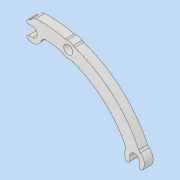
# Autodesk Inventor part: HallEffectSpoolSensorMount3Brace
Saved by Autodesk Inventor 2017.3 (Build 213256000, 256)
## iProperties
Created: 2019-01-08
Part Number: HallEffectSpoolSensorMount3Brace
Material: ABS Plastic
Document SubType Name: Modeling
Designer: Derek Wider
Density: 1.06 g/cm^3
Appearance: Smooth - White
Author: Derek Wider
Autodesk Inventor part; units mm, degrees
ref_plane "YZ Plane" through (0, 0, 0) normal (1, 0, 0) x (0, 1, 0)
ref_plane "XZ Plane" through (0, 0, 0) normal (0, 1, 0) x (-1, 0, 0)
ref_plane "XY Plane" through (0, 0, 0) normal (0, 0, 1) x (1, 0, 0)
sketch "Sketch1" plane through (0, 0, 0) normal (0, 0, 1) x (1, 0, 0)
  line L0 (0, 0) -> (69.850633, 0) construction
  circle A0 centre (0, -41.91) radius 47.625 construction
  arc A1 (0, -1.7145) -> (0, 1.7145) centre (0, 0) ccw
  arc A2 (-2.896046, -1.7145) -> (-2.896046, 1.7145) centre (0, 0) ccw
  line L1 (0, 3.3655) -> (0, 4.6355)
  arc A3 (38.009625, -20.955) -> (34.580625, -20.955) centre (36.295125, -20.955) ccw
  arc A4 (38.009625, -23.997704) -> (34.580625, -23.997704) centre (36.295125, -20.955) ccw
  arc A5 (38.009625, -17.912296) -> (0, 4.6355) centre (2.71264, -34.102694) ccw
  arc A6 (33.341029, -19.091972) -> (3.3655, 0) centre (2.71264, -34.102694) ccw
  line L2 (0, 1.7145) -> (-2.896046, 1.7145)
  line L3 (0, -1.7145) -> (-2.896046, -1.7145)
  line L4 (34.580625, -20.955) -> (34.580625, -23.997704)
  line L5 (38.009625, -20.955) -> (38.009625, -23.997704)
  dimension "d0" = 41.91
  dimension "d2" = 30
  dimension "d3" = 95.25
  dimension "d4" = 41.91
  dimension "d5" = 41.91
  dimension "d6" = 3.429
  dimension "d7" = 6.731
  dimension "d8" = 1.27
  dimension "d9" = 3.429
  dimension "d10" = 6.985
  constraints: 16 point on circle, 12 end point, 7 centre point, 4 coincident, 2 horizontal, 2 parallel, 2 tangent, 2 vertical, 1 concentric, 1 point on line
  measures "d0" distance of point (36.295, -20.955) L0.start
  measures "d3" diameter of A0
  measures "d4" distance of A0.centre L0.start
  measures "d5" distance of A0.centre point (36.295, -20.955)
  measures "d6" diameter of A1
  measures "d7" diameter of A2
  measures "d8" distance of L1.start L1.end
  measures "d9" diameter of A3
  measures "d10" diameter of A4
extrude "Extrusion1" add sketch "Sketch1" along normal blind 3.175
fillet "Fillet1" radius 0.635 4 edges at (-2.896, -1.7145, 1.5875) (-2.896, 1.7145, 1.5875) (34.5806, -23.9977, 1.5875) (38.0096, -23.9977, 1.5875)
fillet "Fillet2" radius 1.778 5 edges at (0, 3.3655, 1.5875) (0, 4.6355, 1.5875) (3.3655, 0, 1.5875) (33.341, -19.092, 1.5875) (38.0096, -17.9123, 1.5875)
sketch "Sketch2" plane through (0, 0, 3.175) normal (0, 0, 1) x (1, 0, 0)
  circle A0 centre (12.7, 0.889) radius 1.5875
  point P0 (0, 0)
  dimension "d15" = 3.175
  dimension "d16" = 12.7
  dimension "d17" = 0.889
  constraints: 1 centre point
  measures "d15" diameter of A0
  measures "d16" horizontal distance of A0.centre point (0, 0)
  measures "d17" vertical distance of A0.centre point (0, 0)
extrude "Extrusion2" cut sketch "Sketch2" against normal through all
sketch "Sketch3" plane through (0, 0, 3.175) normal (0, 0, 1) x (1, 0, 0)
  circle A0 centre (12.7, 0.889) radius 1.5875 projected
  circle A1 centre (12.7, 0.889) radius 2.794
  point P0 (0, 0)
  dimension "d20" = 5.588
  constraints: 1 centre point, 1 coincident
  measures "d20" diameter of A1
extrude "Extrusion3" add sketch "Sketch3" against normal blind 3.175
fillet "Fillet3" radius 1.778 4 edges at (12.019, 3.5987, 1.5875) (14.7087, 2.831, 1.5875) (10.5615, -0.9091, 1.5875) (13.5673, -1.767, 1.5875)
body "Solid1"
